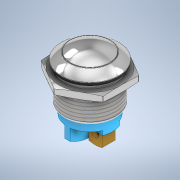
# Autodesk Inventor part: Push Button 16mm
Saved by Autodesk Inventor 2021 (Build 250183000, 183)
## iProperties
Created: 2024-01-18
Part Number: Push Button 16mm
Material: Generic
Document SubType Name: Modeling
Designer: aaronpaulberroya
Density: 1 g/cm^3
Appearance: Default
Author: aaronpaulberroya
Autodesk Inventor part; units mm, degrees
sketch "Sketch2" plane through (0, 0, 0) normal (1, 0, 0) x (0, 1, 0)
  line L0 (0, 0) -> (0, 8.925)
  line L1 (0, 6.025) -> (1.9, 6.025)
  line L2 (0, 0) -> (0.1708, 0)
  line L3 (0.1708, 0) -> (3.6708, 0)
  line L4 (3.6708, 0) -> (0, 8.925)
  line L5 (1.201, 6.005) -> (0, 6.005)
  line L6 (0, 0) -> (-0.2141, 0)
  line L7 (1.201, 6.005) -> (1.201, 0)
  line L8 (1.201, -6.005) -> (1.201, 0)
  line L9 (0, 0) -> (0, -8.925)
  line L10 (3.6708, 0) -> (0, -8.925)
  line L11 (1.201, -6.005) -> (0, -6.005)
  arc A0 (0, -8.925) -> (0, 8.925) centre (-9.0144, 0) ccw
  line L12 (1.1928, 6.025) -> (2.1487, 6.025)
  line L13 (1.201, 6.005) -> (2.1595, 6.005)
  line L14 (0, 7.9) -> (-10, 7.9)
  line L15 (0, 0) -> (-13.7439, 0)
  line L16 (-10, 7.9) -> (-10, 0)
  line L17 (-10, 7.9) -> (-10.9, 7.9)
  line L18 (-11.9, 6.9) -> (-11.9, 0)
  arc A1 (-10.9, 7.9) -> (-11.9, 6.9) centre (-10.9, 6.9) ccw
  point P0 (-11.9, 7.9)
  dimension "d2" = 8.925
  dimension "d4" = 2.9
  dimension "d5" = 3.5
  dimension "d6" = 0.02
  dimension "d7" = 10
  dimension "d8" = 7.9
  dimension "d9" = 1.9
  dimension "d10" = 1
  constraints: 38 end point, 16 point on line, 7 point on circle, 5 horizontal, 4 perpendicular, 3 symmetric about line, 2 centre point, 2 tangent, 1 collinear, 1 vertical
  measures "d2" distance of L0.start L0.end
  measures "d4" distance from line of L0.end L1
  measures "d5" distance of L2.end L3.end
  measures "d6" distance between parallel lines of L5 L1
  measures "d7" distance of L14.start L14.end
  measures "d8" distance of L14.end L16.end
  measures "d9" distance of L14.end point (-11.9, 7.9)
  measures "d10" radius of A1
revolve "Revolution1" add sketch "Sketch2" angle 360 about axis through (0, 0, 0) along (0, -1, 0) contours L6 L15 L16 L14 L0 | L0 L5 L7 L3 L2 | L0 L4 L1 | L13 A0 L4 | L4 L3 L7 | L4 A0 L12 L1
sketch "Sketch3" plane through (0, 0, 0) normal (0, -1, 0) x (1, 0, 0)
  circle A0 centre (0, 0) radius 8.75
  circle A1 centre (0, 0) radius 7.9
  dimension "d12" = 17.5
  dimension "d19" = 15.8
  constraints: 2 centre point, 2 coincident
  measures "d12" diameter of A0
  measures "d19" diameter of A1
extrude "Extrusion1" add sketch "Sketch3" along normal blind 1 separate body
fillet "Fillet1" radius 0.5 2 edges at (-8.75, -1, 0) (-8.75, 0, 0)
fillet "Fillet2" radius 0.1 1 edges at (0, 0, -8.925)
fillet "Fillet3" radius 0.1 2 edges at (0, 2.1487, -6.025) (0, 2.1595, -6.005)
revolve "Revolution2" add sketch "Sketch2" angle 360 about axis through (0, 0, 0) along (0, -1, 0) bodies 1 contours L15 L18 A1 L17 L16
sketch "Sketch4" plane through (0, -11.9, 0) normal (0, -1, 0) x (1, 0, 0)
  circle A0 centre (0, 0) radius 6.9 projected
extrude "Extrusion2" add sketch "Sketch4" along normal blind 7.8 separate body
sketch "Sketch5" plane through (0, 0, 0) normal (1, 0, 0) x (0, 1, 0)
  line L0 (-19.7, 6.9) -> (-19.7, -6.9) projected
  line L1 (-11.9, -6.9) -> (-19.7, -6.9) projected
  line L2 (-17.7, -6.9) -> (-17.7, 6.9)
  line L3 (-11.9, 6.9) -> (-19.7, 6.9) projected
  arc A0 (-17.7, 6.9) -> (-17.7, -6.9) centre (-6.7975, 0) ccw
  line L4 (-19.7, -6.9) -> (-17.7, -6.9)
  line L5 (-17.7, -6.9) -> (-17.7, 6.9)
  line L6 (-17.7, 6.9) -> (-19.7, 6.9)
  line L7 (-19.7, 6.9) -> (-19.7, -6.9)
  point P0 (0, 0)
  point P1 (-19.7, 0)
  dimension "d23" = 2
  constraints: 10 end point, 2 parallel, 2 point on circle, 2 point on line, 1 centre point, 1 horizontal, 1 perpendicular, 1 vertical
  measures "d23" distance between parallel lines of L0 L2
extrude "Extrusion3" cut sketch "Sketch5" along normal mid plane 1.57 contours L3 A0 L0 | A0 L1 L0 bodies 3
ref_plane "Work Plane1" through (0, 0, 9.525) normal (0, 0, 1) x (1, 0, 0)
sketch "Sketch6" plane through (0, 0, 9.525) normal (0, 0, 1) x (1, 0, 0)
  line L0 (0.785, -19.7) -> (6.9, -19.7) projected
  line L1 (-6.9, -11.9) -> (-6.9, -19.7) projected
  line L2 (6.9, -19.7) -> (-6.9, -19.7)
  line L3 (-6.9, -19.7) -> (-6.9, -14.2)
  line L4 (-6.9, -14.2) -> (6.9, -14.2)
  line L5 (6.9, -14.2) -> (6.9, -19.7)
  line L6 (-6.9, -11.9) -> (6.9, -11.9) projected
  line L7 (0.785, -17.7282) -> (0.785, -19.7) projected
  line L8 (0.785, -19.7) -> (6.9, -19.7)
  line L9 (6.9, -19.7) -> (6.9, -14.2)
  line L10 (6.9, -14.2) -> (0.785, -14.2)
  line L11 (0.785, -14.2) -> (0.785, -19.7)
  line L12 (-6.9, -19.7) -> (-0.785, -19.7) projected
  line L13 (-0.785, -19.7) -> (-6.9, -19.7)
  line L14 (-6.9, -19.7) -> (-6.9, -14.2)
  line L15 (-6.9, -14.2) -> (-0.785, -14.2)
  line L16 (-0.785, -14.2) -> (-0.785, -19.7)
  point P0 (0, 0)
  point P1 (0.785, -14.2)
  dimension "d29" = 2.3
  constraints: 24 end point, 6 parallel, 3 horizontal, 3 perpendicular, 1 point on line
  measures "d29" distance between parallel lines of L6 L4
extrude "Extrusion4" cut sketch "Sketch6" against normal through all contours L7 L11 L4 L5 L0 | L2 L1 L4 L16 bodies 3
sketch "Sketch7" plane through (0, -14.2, 0) normal (0, -1, 0) x (1, 0, 0)
  line L0 (1.1914, 2.6) -> (6.3914, 2.6)
  line L1 (6.3914, 2.6) -> (6.3914, -2.6)
  line L2 (6.3914, -2.6) -> (1.1914, -2.6)
  line L3 (1.1914, -2.6) -> (1.1914, 2.6)
  line L4 (1.1914, 2.6) -> (6.3914, -2.6) construction
  line L5 (6.3914, 2.6) -> (1.1914, -2.6) construction
  line L6 (0, 0) -> (9.9463, 0)
  arc A0 (0.785, -6.8552) -> (0.785, 6.8552) centre (0, 0) ccw projected
  point P0 (3.7914, 0)
  dimension "d32" = 5.2
  dimension "d34" = 5.2
  constraints: 14 end point, 2 horizontal, 2 midpoint, 2 parallel, 1 perpendicular, 1 point on circle, 1 point on line
  measures "d32" distance of L1.end L2.end
  measures "d34" distance of L0.end L1.end
extrude "Extrusion5" add sketch "Sketch7" along normal blind 1.3 bodies 3
ref_plane "Work Plane2" through (0, -21.85, 0) normal (0, -1, 0) x (1, 0, 0)
sketch "Sketch8" plane through (0, -15.5, 0) normal (0, -1, 0) x (1, 0, 0)
  line L0 (1.6537, -2) -> (5.6537, -2)
  line L1 (5.6537, -2) -> (5.6537, 2)
  line L2 (5.6537, 2) -> (1.6537, 2)
  line L3 (1.6537, 2) -> (1.6537, -2)
  line L4 (1.6537, -2) -> (5.6537, 2) construction
  line L5 (5.6537, -2) -> (1.6537, 2) construction
  point P0 (0, 0)
  point P1 (3.6537, 0)
  dimension "d37" = 4
  dimension "d38" = 4
  constraints: 12 end point, 2 midpoint, 2 parallel, 1 horizontal, 1 perpendicular
  measures "d37" distance of L2.end L1.end
  measures "d38" distance of L1.end L0.end
extrude "Extrusion6" add sketch "Sketch8" along normal blind 4.2 separate body
sketch "Sketch13" plane through (6.3914, -14.2, -2.6) normal (0, 0, -1) x (-1, 0, 0)
  circle A0 centre (2.7377, -2.3028) radius 1.1
  line L0 (0.7377, -1.3) -> (0.7377, -5.5) projected
  point P0 (6.3914, 14.2)
  dimension "d53" = 2.2
  dimension "d54" = 2
  constraints: 1 centre point
  measures "d53" diameter of A0
  measures "d54" distance from line of L0 A0.centre
extrude "Extrusion10" cut sketch "Sketch13" against normal up to next bodies 3
sketch "Sketch14" plane through (5.6537, -15.5, -2) normal (0, 0, -1) x (-1, 0, 0)
  arc A0 (2.4521, 0) -> (1.5479, 0) centre (2, -1.0028) ccw projected
  circle A1 centre (2, -1.0028) radius 1.1
  point P0 (5.6537, 15.5)
  point P1 (1.5479, 0)
  point P2 (2.4521, 0)
  dimension "d57" = 2.2
  constraints: 1 centre point, 1 coincident
  measures "d57" diameter of A1
extrude "Extrusion11" cut sketch "Sketch14" against normal through all bodies 4
sketch "Sketch15" plane through (0, -19.7, 0) normal (0, -1, 0) x (1, 0, 0)
  circle A0 centre (3.6537, 0) radius 1.1
  line L0 (5.6537, 2) -> (1.6537, 2) projected
  line L1 (5.6537, -2) -> (5.6537, 2) projected
  point P0 (0, 0)
  dimension "d60" = 2.2
  dimension "d61" = 2
  dimension "d62" = 2
  constraints: 1 centre point
  measures "d60" diameter of A0
  measures "d61" distance from line of L0 A0.centre
  measures "d62" distance from line of L1 A0.centre
extrude "Extrusion12" cut sketch "Sketch15" against normal up to next bodies 4
sketch "Sketch16" plane through (5.6537, -19.7, -2) normal (0, 0, -1) x (-1, 0, 0)
  line L0 (4, 0) -> (0, 0) projected
  line L1 (0, 4.2) -> (0, 0) projected
  line L2 (4, 0) -> (0, 0)
  line L3 (0, 0) -> (0, 0.3)
  line L4 (0, 0.3) -> (4, 0.3)
  line L5 (4, 0.3) -> (4, 0)
  arc A0 (0, 0.3) -> (4, 0.3) centre (2, 6.8167) ccw
  point P0 (5.6537, 19.7)
  point P1 (2, 0)
  dimension "d65" = 0.3
  constraints: 8 end point, 2 parallel, 2 point on circle, 1 centre point, 1 horizontal, 1 perpendicular, 1 point on line, 1 tangent
  measures "d65" distance between parallel lines of L0 L4
extrude "Extrusion13" cut sketch "Sketch16" against normal blind 4.2 contours L0 A0 L5 | L0 L1 A0 bodies 4
mirror "Mirror2" about plane through (0, 0, 0) normal (1, 0, 0) of "Extrusion6", "Extrusion11", "Extrusion12", "Extrusion13" bodies 4
mirror "Mirror3" about plane through (0, 0, 0) normal (1, 0, 0) of "Extrusion5" bodies 3
ref_plane "Work Plane4" through (0, -2, 0) normal (0, -1, 0) x (1, 0, 0)
sketch "Sketch18" plane through (0, -2, 0) normal (0, -1, 0) x (1, 0, 0)
  line L0 (0, -10.9119) -> (-9.45, -5.456)
  line L1 (-9.45, -5.456) -> (-9.45, 5.456)
  line L2 (-9.45, 5.456) -> (0, 10.9119)
  line L3 (0, 10.9119) -> (9.45, 5.456)
  line L4 (9.45, 5.456) -> (9.45, -5.456)
  line L5 (9.45, -5.456) -> (0, -10.9119)
  circle A0 centre (0, 0) radius 7.9
  dimension "d69" = 18.9
  constraints: 12 end point, 2 coincident, 1 centre point, 13 other
  measures "d69" distance between parallel lines of L1 L4
extrude "Extrusion14" add sketch "Sketch18" along normal blind 2.6 separate body
sketch "Sketch20" plane through (0, -2, 0) normal (0, 1, 0) x (1, 0, 0)
  circle A0 centre (0, 0) radius 9.45
  line L0 (0, -10.9119) -> (-9.45, -5.456) projected
  line L1 (9.45, 5.456) -> (9.45, -5.456) projected
  line L2 (0, 10.9119) -> (9.45, 5.456) projected
  line L3 (-9.45, 5.456) -> (0, 10.9119) projected
  line L4 (-9.45, -5.456) -> (-9.45, 5.456) projected
  line L5 (0, -10.9119) -> (-9.45, -5.456) projected
  line L6 (9.45, -5.456) -> (0, -10.9119) projected
  circle A1 centre (0, 0) radius 7.9 projected
  constraints: 1 centre point, 1 coincident, 1 tangent
extrude "Extrusion15" cut sketch "Sketch20" against normal blind 2 draft 80 contours A0 | A1 keep common part bodies 5
chamfer "Chamfer1" distance 0.2 angle 45 1 edges at (-7.9, -2, 0)
fillet "Fillet4" radius 0.2 6 edges at (9.45, -3.1289, 5.456) (9.45, -3.1289, -5.456) (0, -3.1289, -10.9119) (-9.45, -3.1289, -5.456) (-9.45, -3.1289, 5.456) (0, -3.1289, 10.9119)
sketch "Sketch21" plane through (0, -4, 0) normal (0, -1, 0) x (1, 0, 0)
  circle A0 centre (0, 0) radius 9.45
  constraints: 1 centre point, 1 coincident
extrude "Extrusion16" cut sketch "Sketch21" against normal blind 2 draft 80 keep common part bodies 5
chamfer "Chamfer2" distance 0.2 angle 45 1 edges at (-7.9, -4, 0)
thread "Thread1" size "M16x1" class "6g" standard "ANSI Metric M Profile" full length
body "Solid1"
body "Solid2"
body "Solid3"
body "Solid4"
body "Solid5"
